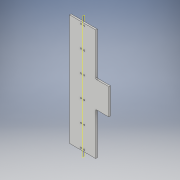
# Autodesk Inventor part: Backhoe to Frame Mount
Saved by Autodesk Inventor 2019 (Build 230136000, 136)
## iProperties
Created: 2018-11-29
Part Number: Backhoe to Frame Mount
Material: Generic
Document SubType Name: Modeling
Designer: Alex Barnett
Density: 1 g/cm^3
Appearance: Default
Author: Alex Barnett
Autodesk Inventor part; units mm, degrees
ref_plane "YZ Plane" through (0, 0, 0) normal (1, 0, 0) x (0, 1, 0)
ref_plane "XZ Plane" through (0, 0, 0) normal (0, 1, 0) x (-1, 0, 0)
ref_plane "XY Plane" through (0, 0, 0) normal (0, 0, 1) x (1, 0, 0)
sketch "Sketch1" plane through (0, 0, 0) normal (0, 0, 1) x (1, 0, 0)
  line L0 (0, 0) -> (101.6, 0)
  line L1 (101.6, 0) -> (101.6, 431.8)
  line L2 (101.6, 431.8) -> (0, 431.8)
  line L3 (0, 431.8) -> (0, 0)
  dimension "d0" = 101.6
  dimension "d1" = 431.8
  constraints: 8 end point, 2 parallel, 1 horizontal, 1 perpendicular
  measures "d0" distance of L2.end L1.end
  measures "d1" distance of L1.end L0.end
extrude "Extrusion1" add sketch "Sketch1" against normal blind 6.35
sketch "Sketch2" plane through (0, 0, 0) normal (0, 0, 1) x (1, 0, 0)
  line L0 (101.6, 0) -> (101.6, 431.8) projected
  line L1 (101.6, 266.7) -> (152.4, 266.7)
  line L2 (152.4, 266.7) -> (152.4, 165.1)
  line L3 (152.4, 165.1) -> (101.6, 165.1)
  line L4 (101.6, 165.1) -> (101.6, 266.7)
  point P0 (0, 0)
  point P1 (101.6, 215.9)
  point P2 (101.6, 215.9)
  dimension "d4" = 50.8
  dimension "d5" = 101.6
  dimension "d6" = 50.8
  constraints: 8 end point, 2 midpoint, 2 parallel, 1 horizontal, 1 perpendicular
  measures "d4" distance of L2.end L3.end
  measures "d5" distance of L1.end L2.end
  measures "d6" distance from line of L2 point (101.6, 215.9)
extrude "Extrusion2" add sketch "Sketch2" against normal blind 6.35
fillet "Fillet1" radius 3.175 1 edges at (101.6, 266.7, -3.175)
fillet "Fillet2" radius 3.175 1 edges at (101.6, 165.1, -3.175)
sketch "Sketch3" plane through (0, 0, 0) normal (0, 0, 1) x (1, 0, 0)
  line L0 (101.6, 0) -> (101.6, 161.925) projected
  line L1 (0, 0) -> (101.6, 0) projected
  point P0 (44.45, 7.62)
  dimension "d11" = 57.15
  dimension "d12" = 7.62
  measures "d11" distance from line of L0 point (44.45, 7.62)
  measures "d12" distance from line of L1 point (44.45, 7.62)
hole "Hole1" at (44.45, 7.62, 0) direction (0, 0, -1) diameter 5.08 end through all
ref_plane "Work Plane1" through (50.8, 0, 0) normal (-1, 0, 0) x (0, 0, 1)
pattern_linear "Rectangular Pattern1" count 2 spacing 12.7 along (1, 0, 0) count 6 spacing 83.312 along (0, 1, 0) of "Hole1"
body "Solid1"
